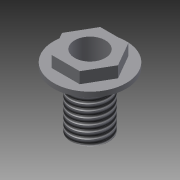
# Autodesk Inventor part: TUNING PEG RETAINER
Saved by Autodesk Inventor 2013 (Build 170138000, 138)
## iProperties
Created: 2014-06-22
Part Number: TUNING PEG RETAINER
Material: Generic
Document SubType Name: Modeling
Designer: employee
Density: 1 g/cm^3
Author: employee
Autodesk Inventor part; units mm, degrees
ref_plane "YZ Plane" through (0, 0, 0) normal (1, 0, 0) x (0, 1, 0)
ref_plane "XZ Plane" through (0, 0, 0) normal (0, 1, 0) x (-1, 0, 0)
ref_plane "XY Plane" through (0, 0, 0) normal (0, 0, 1) x (1, 0, 0)
sketch "Sketch1" plane through (0, 0, 0) normal (0, 0, 1) x (1, 0, 0)
  circle A0 centre (0, 0) radius 3.85
  circle A1 centre (0, 0) radius 3.125
  dimension "d0" = 7.7
  dimension "d2" = 6.25
  constraints: 2 centre point, 2 coincident
  measures "d0" diameter of A0
  measures "d2" diameter of A1
extrude "Extrusion1" add sketch "Sketch1" along normal blind 14.45
sketch "Sketch2" plane through (0, 0, 14.45) normal (0, 0, 1) x (1, 0, 0)
  circle A0 centre (0, 0) radius 3.85 projected
  line L0 (-2.8579, 4.95) -> (2.8579, 4.95)
  line L1 (2.8579, 4.95) -> (5.7158, 0)
  line L2 (5.7158, 0) -> (2.8579, -4.95)
  line L3 (2.8579, -4.95) -> (-2.8579, -4.95)
  line L4 (-2.8579, -4.95) -> (-5.7158, 0)
  line L5 (-5.7158, 0) -> (-2.8579, 4.95)
  dimension "d5" = 9.9
  constraints: 12 end point, 1 coincident, 1 horizontal, 13 other
  measures "d5" distance between parallel lines of L3 L0
extrude "Extrusion2" add sketch "Sketch2" against normal blind 2.3
sketch "Sketch3" plane through (0, 0, 12.15) normal (0, 0, -1) x (-1, 0, 0)
  circle A0 centre (0, 0) radius 3.85 projected
  circle A1 centre (0, 0) radius 7.4
  dimension "d8" = 14.8
  constraints: 1 centre point, 1 coincident
  measures "d8" diameter of A1
extrude "Extrusion3" add sketch "Sketch3" along normal blind 1
thread "Thread1" size "M8x1.25" class "6g" standard "ANSI Metric M Profile" full length
body "Solid1"
